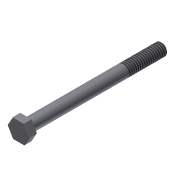
# Autodesk Inventor part: 375 bolt x4
Saved by Autodesk Inventor 2011 (Build 150239000, 239)
## iProperties
Created: 2011-07-05
Part Number: 375 bolt x4
Document SubType Name: Modeling
Designer: Dan Niemitalo
Density: 7.85 g/cm^3
Material: Steel
Mass: 40.1249 g
Surface Area: 26.9431 cm^2
Volume: 5.11145 cm^3
Author: Dan Niemitalo
Autodesk Inventor part; units mm, degrees
ref_plane "YZ Plane" through (0, 0, 0) normal (1, 0, 0) x (0, 1, 0)
ref_plane "XZ Plane" through (0, 0, 0) normal (0, 1, 0) x (-1, 0, 0)
ref_plane "XY Plane" through (0, 0, 0) normal (0, 0, 1) x (1, 0, 0)
sketch "Sketch1" plane through (0, 0, 0) normal (0, 0, 1) x (1, 0, 0)
  circle A0 centre (0, 0) radius 3.9688
  dimension "d0" = 7.9375
  constraints: 1 centre point, 1 coincident
  measures "d0" diameter of A0
extrude "Extrusion1" add sketch "Sketch1" against normal blind 88.9
sketch "Sketch2" plane through (0, 0, 0) normal (0, 0, 1) x (1, 0, 0)
  circle A0 centre (0, 0) radius 3.9687 projected
  line L0 (-7.3323, 0) -> (-3.6662, 6.35)
  line L1 (-3.6662, 6.35) -> (3.6662, 6.35)
  line L2 (3.6662, 6.35) -> (7.3323, 0)
  line L3 (7.3323, 0) -> (3.6662, -6.35)
  line L4 (3.6662, -6.35) -> (-3.6662, -6.35)
  line L5 (-3.6662, -6.35) -> (-7.3323, 0)
  dimension "d3" = 12.7
  constraints: 12 end point, 1 coincident, 13 other
  measures "d3" distance between parallel lines of L4 L1
extrude "Extrusion2" add sketch "Sketch2" along normal blind 5.1594 contours A0 | L0 L1 L2 L3 L4 L5
thread "Thread1" size "5/16-18 UNC" class "2A" standard "ANSI Unified Screw Threads" length 25.4
chamfer "Chamfer1" distance 0.508 angle 45 1 edges at (-3.9688, 0, -88.9)
fillet "Fillet1" radius 0.508 18 edges at (0, 6.35, 5.1594) (-5.4993, 3.175, 5.1594) (-5.4993, -3.175, 5.1594) (0, -6.35, 5.1594) (5.4993, -3.175, 5.1594) (5.4993, 3.175, 5.1594) (-5.4993, 3.175, 0) (0, 6.35, 0) (5.4993, 3.175, 0) (5.4993, -3.175, 0) (0, -6.35, 0) (-5.4993, -3.175, 0) (7.3323, 0, 2.5797) (3.6662, -6.35, 2.5797) (3.6662, 6.35, 2.5797) (-3.6662, -6.35, 2.5797) (-7.3323, 0, 2.5797) (-3.6662, 6.35, 2.5797)
body "Solid1"
